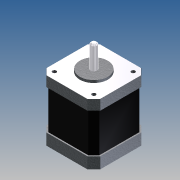
# Autodesk Inventor part: PM Wantai 811  Nema 17
Saved by Autodesk Inventor 2015 (Build 190159000, 159)
## iProperties
Created: 2013-09-15
Part Number: PM Wantai 811  Nema 17
Document SubType Name: Modeling
Designer: Phil
Density: 1 g/cm^3
Material: Generic
Appearance: Aluminum Cast
Author: Phil
Autodesk Inventor part; units mm, degrees
ref_plane "YZ Plane" through (0, 0, 0) normal (1, 0, 0) x (0, 1, 0)
ref_plane "XZ Plane" through (0, 0, 0) normal (0, 1, 0) x (-1, 0, 0)
sketch "Sketch1" plane through (0, 0, 0) normal (0, 0, 1) x (1, 0, 0)
  line L0 (-21.15, 21.15) -> (21.15, 21.15)
  line L1 (21.15, 21.15) -> (21.15, -21.15)
  line L2 (21.15, -21.15) -> (-21.15, -21.15)
  line L3 (-21.15, -21.15) -> (-21.15, 21.15)
  point P0 (0, 0)
  dimension "d0" = 42.3
  dimension "d1" = 42.3
  dimension "d2" = 21.15
  dimension "d3" = 21.15
  constraints: 8 end point, 2 parallel, 1 horizontal, 1 perpendicular
  measures "d0" distance between parallel lines of L2 L0
  measures "d1" distance of L1.end L2.end
  measures "d2" distance from line of L3 point (0, 0)
  measures "d3" distance from line of L2 point (0, 0)
extrude "Extrusion1" add sketch "Sketch1" along normal blind 48
sketch "Sketch2" plane through (0, 0, 48) normal (0, 0, 1) x (1, 0, 0)
  circle A0 centre (0, 0) radius 11
  dimension "d6" = 22
  constraints: 1 centre point, 1 coincident
  measures "d6" diameter of A0
extrude "Extrusion2" add sketch "Sketch2" along normal blind 2
sketch "Sketch3" plane through (0, 0, 50) normal (0, 0, 1) x (1, 0, 0)
  circle A0 centre (0, 0) radius 11 projected
  circle A1 centre (0, 0) radius 2.5
  dimension "d9" = 5
  constraints: 1 centre point, 1 coincident
  measures "d9" diameter of A1
extrude "Extrusion3" add sketch "Sketch3" along normal blind 18 contours A1
chamfer "Chamfer1" distance 5 angle 45 4 edges at (-21.15, 21.15, 24) (21.15, 21.15, 24) (-21.15, -21.15, 24) (21.15, -21.15, 24)
ref_plane "Work Plane1" through (0, 0, 40) normal (0, 0, 1) x (1, 0, 0)
sketch "Sketch4" plane through (0, 0, 40) normal (0, 0, 1) x (1, 0, 0)
  line L0 (21.15, -16.15) -> (16.15, -21.15) projected
  line L1 (21.15, 16.15) -> (21.15, -16.15) projected
  line L2 (16.15, 21.15) -> (21.15, 16.15) projected
  line L3 (-16.15, 21.15) -> (16.15, 21.15) projected
  line L4 (-21.15, 16.15) -> (-16.15, 21.15) projected
  line L5 (-21.15, -16.15) -> (-21.15, 16.15) projected
  line L6 (-16.15, -21.15) -> (-21.15, -16.15) projected
  line L7 (16.15, -21.15) -> (-16.15, -21.15) projected
  circle A0 centre (0, 0) radius 11 projected
  line L8 (15.7358, 20.15) -> (20.15, 15.7358)
  line L9 (20.15, 15.7358) -> (20.15, -15.7358)
  line L10 (20.15, -15.7358) -> (15.7358, -20.15)
  line L11 (15.7358, -20.15) -> (-15.7358, -20.15)
  line L12 (-15.7358, -20.15) -> (-20.15, -15.7358)
  line L13 (-20.15, -15.7358) -> (-20.15, 15.7358)
  line L14 (-20.15, 15.7358) -> (-15.7358, 20.15)
  line L15 (-15.7358, 20.15) -> (15.7358, 20.15)
  dimension "d16" = 1
  constraints: 16 end point, 7 other
  measures "d16" distance between parallel lines of L15 L3
extrude "Extrusion4" cut sketch "Sketch4" against normal blind 31 contours L0 L7 L6 L5 L4 L3 L2 L1
sketch "Sketch5" plane through (0, 0, 48) normal (0, 0, 1) x (1, 0, 0)
  line L0 (16.15, -21.15) -> (-16.15, -21.15) projected
  circle A0 centre (0, 0) radius 11 projected
  line L1 (0, 0) -> (0, 35.0575) construction
  line L2 (0, 0) -> (-35.907, 0) construction
  circle A1 centre (-15.5, 15.5) radius 1.5
  circle A2 centre (15.5, 15.5) radius 1.5
  circle A3 centre (-15.5, -15.5) radius 1.5
  circle A4 centre (15.5, -15.5) radius 1.5
  dimension "d19" = 3
  dimension "d20" = 15.5
  dimension "d21" = 15.5
  constraints: 4 centre point, 4 end point, 3 symmetric about line, 2 perpendicular, 3 other
  measures "d19" diameter of A1
  measures "d20" distance from line of L1 A1.centre
  measures "d21" distance from line of L2 A1.centre
extrude "Extrusion5" cut sketch "Sketch5" against normal blind 4 contours A1 | A2 | A3 | A4
fillet "Fillet1" radius 0.1 16 edges at (18.65, -18.65, 48) (21.15, 0, 48) (18.65, 18.65, 48) (0, 21.15, 48) (-18.65, 18.65, 48) (-21.15, 0, 48) (-18.65, -18.65, 48) (0, -21.15, 48) (18.65, -18.65, 0) (0, -21.15, 0) (-18.65, -18.65, 0) (-21.15, 0, 0) (-18.65, 18.65, 0) (0, 21.15, 0) (18.65, 18.65, 0) (21.15, 0, 0)
chamfer "Chamfer2" distance 1 angle 45 1 edges at (-2.5, 0, 68)
thread "Thread1" size "M3x0.5" class "6H" standard "ANSI Metric M Profile" full length
thread "Thread2" size "M3x0.5" class "6H" standard "ANSI Metric M Profile" full length
thread "Thread3" size "M3x0.5" class "6H" standard "ANSI Metric M Profile" full length
thread "Thread4" size "M3x0.5" class "6H" standard "ANSI Metric M Profile" full length
sketch "Sketch7" plane through (0, 0, 0) normal (0, 0, -1) x (-1, 0, 0)
  line L0 (0, 0) -> (30.0601, 0) construction
  line L1 (21.05, 16.1086) -> (21.05, -16.1086) projected
  line L2 (21.15, -16.15) -> (21.15, 16.15) projected
  line L3 (25.65, 8.15) -> (21.05, 8.15)
  line L4 (21.05, 8.15) -> (21.05, -8.15)
  line L5 (21.05, -8.15) -> (25.65, -8.15)
  line L6 (25.65, -8.15) -> (25.65, 8.15)
  dimension "d38" = 16.3
  dimension "d39" = 8.15
  dimension "d40" = 4.5
  constraints: 10 end point, 2 horizontal, 2 parallel, 1 perpendicular, 1 point on line
  measures "d38" distance between parallel lines of L5 L3
  measures "d39" distance between parallel lines of L0 L3
  measures "d40" distance between parallel lines of L2 L6
extrude "Extrusion7" add sketch "Sketch7" against normal blind 3
sketch "Sketch8" plane through (-21.15, -16.15, 9) normal (-1, 0, 0) x (0, 0, 1)
  line L0 (-6, 24.3) -> (-6, 8) projected
  line L1 (0, 0) -> (0, 32.3) projected
  line L2 (-6, 8) -> (0, 8)
  line L3 (0, 8) -> (0, 24.3)
  line L4 (0, 24.3) -> (-6, 24.3)
  line L5 (-6, 24.3) -> (-6, 8)
  line L6 (-8.9, 24.3) -> (-6, 24.3) projected
  point P0 (-9, 16.15)
  constraints: 8 end point, 2 collinear, 2 parallel, 1 horizontal, 1 perpendicular
extrude "Extrusion8" cut sketch "Sketch8" against normal blind 1
sketch "Sketch9" plane through (-20.15, -15.7358, 40) normal (-1, 0, 0) x (0, 0, 1)
  line L0 (-37, 7.5858) -> (-31, 7.5858)
  line L1 (-31, 7.5858) -> (-31, 23.8858)
  line L2 (-31, 23.8858) -> (-37, 23.8858)
  line L3 (-37, 23.8858) -> (-37, 7.5858)
  point P0 (-40, 15.7358)
  constraints: 8 end point, 2 parallel, 1 horizontal, 1 perpendicular
extrude "Extrusion9" add sketch "Sketch9" along normal blind 7
sketch "Sketch10" plane through (-27.15, -15.7358, 40) normal (-1, 0, 0) x (0, 0, 1)
  line L0 (-37, 7.5858) -> (-31, 7.5858) projected
  line L1 (-31, 7.5858) -> (-31, 23.8858) projected
  line L2 (-31, 23.8858) -> (-37, 23.8858) projected
  line L3 (-37, 23.8858) -> (-37, 7.5858) projected
  line L4 (-36.4, 8.1858) -> (-31.6, 8.1858)
  line L5 (-31.6, 8.1858) -> (-31.6, 23.2858)
  line L6 (-31.6, 23.2858) -> (-36.4, 23.2858)
  line L7 (-36.4, 23.2858) -> (-36.4, 8.1858)
  point P0 (-40, 15.7358)
  dimension "d47" = 0.6
  constraints: 8 end point, 3 other
  measures "d47" distance between parallel lines of L3 L7
extrude "Extrusion10" cut sketch "Sketch10" against normal blind 4.75 contours L7 L6 L5 L4
sketch "Sketch11" plane through (0, 0, 9) normal (0, 0, 1) x (1, 0, 0)
  line L0 (-20.15, 15.7358) -> (-20.15, -15.7358) projected
  line L1 (-15.7358, 20.15) -> (-20.15, 15.7358) projected
  line L2 (15.7358, 20.15) -> (-15.7358, 20.15) projected
  line L3 (20.15, 15.7358) -> (15.7358, 20.15) projected
  line L4 (20.15, -15.7358) -> (20.15, 15.7358) projected
  line L5 (15.7358, -20.15) -> (20.15, -15.7358) projected
  line L6 (-15.7358, -20.15) -> (15.7358, -20.15) projected
  line L7 (-20.15, -15.7358) -> (-15.7358, -20.15) projected
  line L8 (-21.15, 8.15) -> (-27.15, 8.15) projected
  line L9 (-27.15, -8.15) -> (-27.15, 8.15) projected
  line L10 (-21.15, -8.15) -> (-27.15, -8.15) projected
  line L11 (-21.15, -16.15) -> (-21.15, -8.15) projected
  line L12 (-16.15, -21.15) -> (-21.15, -16.15) projected
  line L13 (16.15, -21.15) -> (-16.15, -21.15) projected
  line L14 (21.15, -16.15) -> (16.15, -21.15) projected
  line L15 (21.15, 16.15) -> (21.15, -16.15) projected
  line L16 (16.15, 21.15) -> (21.15, 16.15) projected
  line L17 (-16.15, 21.15) -> (16.15, 21.15) projected
  line L18 (-21.15, 16.15) -> (-16.15, 21.15) projected
  line L19 (-21.15, 8.15) -> (-21.15, 16.15) projected
  line L20 (-27.15, -8.15) -> (-27.15, 8.15) projected
  line L21 (-27.15, 0) -> (-20.15, 0) construction
  line L22 (-20.15, 15.7358) -> (-20.15, -15.7358) projected
  line L23 (-27.15, -4) -> (-22.87, -4)
  line L24 (-22.87, -4) -> (-22.87, 4)
  line L25 (-22.87, 4) -> (-27.15, 4)
  line L26 (-27.15, 4) -> (-27.15, -4)
  point P0 (0, 0)
  dimension "d50" = 8
  dimension "d51" = 4
  dimension "d52" = 4.28
  constraints: 10 end point, 2 midpoint, 2 parallel, 1 horizontal, 1 perpendicular, 1 point on line
  measures "d50" distance between parallel lines of L25 L23
  measures "d51" distance between parallel lines of L21 L23
  measures "d52" distance between parallel lines of L24 L9
extrude "Extrusion11" cut sketch "Sketch11" against normal blind 1 contours L25 L24 L23 L9
sketch "Sketch12" plane through (-25.65, 8.15, 0) normal (0, 1, 0) x (1, 0, 0)
  line L0 (4.5, -0.1) -> (4.5, -9) projected
  line L1 (0, -3) -> (4.5, -3)
  line L2 (4.5, -3) -> (4.5, -3.1)
  line L3 (4.5, -3.1) -> (0, -3.1)
  line L4 (0, -3.1) -> (0, -3)
  point P0 (25.65, 0)
  dimension "d55" = 0.1
  constraints: 8 end point, 2 parallel, 1 horizontal, 1 perpendicular, 1 point on line
  measures "d55" distance between parallel lines of L1 L3
extrude "Extrusion12" cut sketch "Sketch12" against normal blind 0.1
mirror "Mirror1" about plane through (0, 0, 0) normal (0, 1, 0) of "Extrusion12"
sketch "Sketch13" plane through (0, 0, 9) normal (0, 0, 1) x (1, 0, 0)
  line L0 (-20.15, 15.7358) -> (-20.15, -15.7358) projected
  line L1 (-20.15, 8.15) -> (-20.15, 8.05)
  line L2 (-21.15, 8.15) -> (-21.15, 16.15) projected
  line L3 (-21.15, 8.2) -> (-20.15, 8.2)
  line L4 (-20.15, 8.2) -> (-20.15, 8.1)
  line L5 (-20.15, 8.1) -> (-21.15, 8.1)
  line L6 (-21.15, 8.1) -> (-21.15, 8.2)
  point P0 (0, 0)
  dimension "d61" = 0.1
  dimension "d62" = 0.05
  constraints: 10 end point, 3 point on line, 2 parallel, 1 horizontal, 1 perpendicular
  measures "d61" distance between parallel lines of L3 L5
  measures "d62" distance from line of L5 L2.start
extrude "Extrusion13" cut sketch "Sketch13" against normal blind 0.1
mirror "Mirror2" about plane through (0, 0, 0) normal (0, 1, 0) of "Extrusion13"
sketch "Sketch14" plane through (-22.4, -15.7358, 40) normal (-1, 0, 0) x (0, 0, 1)
  line L0 (-31.6, 8.1858) -> (-36.4, 8.1858) projected
  line L1 (-31.6, 23.2858) -> (-31.6, 8.1858) projected
  line L2 (-36.4, 23.2858) -> (-31.6, 23.2858) projected
  line L3 (-36.4, 8.1858) -> (-36.4, 23.2858) projected
  line L4 (-36.4, 8.1858) -> (-36.4, 23.2858) projected
  line L5 (-36.4, 15.7358) -> (-31.6, 15.7358) construction
  line L6 (-34.25, 14.4858) -> (-33.75, 14.4858)
  line L7 (-33.75, 14.4858) -> (-33.75, 14.9858)
  line L8 (-33.75, 14.9858) -> (-34.25, 14.9858)
  line L9 (-34.25, 14.9858) -> (-34.25, 14.4858)
  line L10 (-34, 15.7358) -> (-34, 8.6812) construction
  point P0 (-40, 15.7358)
  dimension "d63" = 0.75
  dimension "d64" = 0.5
  dimension "d65" = 0.25
  dimension "d66" = 0.5
  constraints: 12 end point, 3 midpoint, 2 horizontal, 2 parallel, 1 perpendicular, 1 vertical
  measures "d63" distance between parallel lines of L5 L8
  measures "d64" distance between parallel lines of L7 L9
  measures "d65" distance between parallel lines of L10 L9
  measures "d66" distance between parallel lines of L8 L6
extrude "Extrusion14" add sketch "Sketch14" along normal blind 4.6 contours L9 L8 L7 L6
chamfer "Chamfer3" distance 0.08 angle 70 4 edges at (-27, -1, 6.25) (-27, -0.75, 6) (-27, -1, 5.75) (-27, -1.25, 6) measured on face at (-27, -0.9167, 5.9167)
pattern_linear "Rectangular Pattern1" count 3 spacing 2.5 along (0, -1, 0) of "Extrusion14", "Chamfer3"
mirror "Mirror3" about plane through (0, 0, 0) normal (0, 1, 0) of "Extrusion14", "Chamfer3", "Rectangular Pattern1"
sketch "Sketch15" plane through (0, 0, 0) normal (0, 0, -1) x (-1, 0, 0)
  circle A0 centre (0, 0) radius 4.595
  dimension "d75" = 9.19
  constraints: 1 centre point, 1 coincident
  measures "d75" diameter of A0
extrude "Extrusion15" cut sketch "Sketch15" against normal blind 3.55
sketch "Sketch16" plane through (0, 0, 0) normal (0, 0, -1) x (-1, 0, 0)
  circle A0 centre (0, 0) radius 4.595 projected
  line L0 (21.05, 16.1086) -> (21.05, 8.15) projected
  line L1 (16.1086, 21.05) -> (21.05, 16.1086) projected
  line L2 (-16.1086, 21.05) -> (16.1086, 21.05) projected
  line L3 (-21.05, 16.1086) -> (-16.1086, 21.05) projected
  line L4 (-21.05, -16.1086) -> (-21.05, 16.1086) projected
  line L5 (-16.1086, -21.05) -> (-21.05, -16.1086) projected
  line L6 (16.1086, -21.05) -> (-16.1086, -21.05) projected
  line L7 (21.05, -16.1086) -> (16.1086, -21.05) projected
  line L8 (21.05, -8.15) -> (21.05, -16.1086) projected
  line L9 (21.05, -8.15) -> (25.65, -8.15) projected
  line L10 (25.65, -8.15) -> (25.65, 8.15) projected
  line L11 (25.65, 8.15) -> (21.05, 8.15) projected
  circle A1 centre (15, 15) radius 3
  dimension "d78" = 15
  dimension "d79" = 15
  dimension "d80" = 6
  constraints: 1 centre point
  measures "d78" horizontal distance of point (0, 0) A1.centre
  measures "d79" horizontal distance of point (0, 0) A1.centre
  measures "d80" diameter of A1
extrude "Extrusion16" cut sketch "Sketch16" against normal blind 2 contours A1
mirror "Mirror4" about plane through (0, 0, 0) normal (1, 0, 0) of "Extrusion16"
mirror "Mirror5" about plane through (0, 0, 0) normal (0, 1, 0) of "Extrusion16", "Mirror4"
sketch "Sketch17" plane through (-15, 15, 2) normal (0, 0, -1) x (-1, 0, 0)
  circle A0 centre (0, 0) radius 3 projected
  circle A1 centre (0, 0) radius 2.45
  point P0 (-15, -15)
  constraints: 1 centre point, 1 coincident
extrude "Extrusion17" add sketch "Sketch17" along normal blind 1.7 contours A1
sketch "Sketch18" plane through (-15, 15, 0.3) normal (0, 0, -1) x (-1, 0, 0)
  circle A0 centre (0, 0) radius 2.45 projected
  line L0 (1.5, 0.5) -> (-1.5, 0.5)
  line L1 (-1.5, 0.5) -> (-1.5, -0.5)
  line L2 (-1.5, -0.5) -> (1.5, -0.5)
  line L3 (1.5, -0.5) -> (1.5, 0.5)
  line L4 (0.5, 1.5) -> (-0.5, 1.5)
  line L5 (-0.5, 1.5) -> (-0.5, -1.5)
  line L6 (-0.5, -1.5) -> (0.5, -1.5)
  line L7 (0.5, -1.5) -> (0.5, 1.5)
  point P0 (-15, -15)
  dimension "d85" = 1
  dimension "d86" = 1
  dimension "d87" = 1.5
  dimension "d88" = 1.5
  dimension "d89" = 1.5
  dimension "d90" = 1.5
  dimension "d91" = 0.5
  dimension "d92" = 0.5
  constraints: 16 end point, 4 parallel, 2 horizontal, 2 perpendicular
  measures "d85" distance between parallel lines of L2 L0
  measures "d86" distance between parallel lines of L5 L7
  measures "d87" distance from line of A0.centre L4
  measures "d88" distance from line of A0.centre L6
  measures "d89" distance from line of A0.centre L3
  measures "d90" distance from line of L1 A0.centre
  measures "d91" distance from line of A0.centre L7
  measures "d92" distance from line of A0.centre L0
extrude "Extrusion18" cut sketch "Sketch18" against normal blind 0.6 contours L3 L2 L7 L0 | L7 L2 L5 L0 | L0 L5 L4 L7 | L5 L2 L1 L0 | L7 L6 L5 L2
fillet "Fillet2" radius 0.5 1 edges at (-12.55, 15, 0.3)
mirror "Mirror6" about plane through (0, 0, 0) normal (1, 0, 0) of "Extrusion17", "Extrusion18", "Fillet2"
mirror "Mirror7" about plane through (0, 0, 0) normal (0, 1, 0) of "Extrusion17", "Extrusion18", "Fillet2", "Mirror6"
sketch "Sketch19" plane through (0, 0, 3.55) normal (0, 0, -1) x (-1, 0, 0)
  circle A0 centre (0, 0) radius 2.5
  circle A1 centre (0, 0) radius 4.595 projected
  circle A2 centre (0, 0) radius 0.2846
  dimension "d96" = 5
  constraints: 2 centre point, 2 coincident
  measures "d96" diameter of A0
extrude "Extrusion19" add sketch "Sketch19" along normal blind 0.6 contours A0
chamfer "Chamfer4" distance 0.2 angle 45 1 edges at (2.5, 0, 2.95)
sketch "Sketch20" plane through (0, 0, 68) normal (0, 0, 1) x (1, 0, 0)
  circle A0 centre (0, 0) radius 2.5 projected
  line L0 (-7.2134, -5.8829) -> (-2, -5.8829)
  line L1 (-2, -5.8829) -> (-2, 8.324)
  line L2 (-2, 8.324) -> (-7.2134, 8.324)
  line L3 (-7.2134, 8.324) -> (-7.2134, -5.8829)
  dimension "d102" = 2
  constraints: 8 end point, 2 parallel, 1 horizontal, 1 perpendicular
  measures "d102" distance from line of L1 point (0, 0)
extrude "Extrusion20" cut sketch "Sketch20" against normal blind 17 contours L1 A0 | A0 L1 L0 L3 L2 picked at (-2.1667, 0)
equation "\"d1\" = d0"
equation "\"d2\" = 0.5 * d1"
equation "\"d3\" = 0.5 * d0"
equation "\"d20\" = d21"
equation "\"d39\" = 0.5 * d38"
equation "\"d51\" = 0.5 * d50"
equation "\"d65\" = 0.5 * d64"
equation "\"d66\" = d64"
equation "\"d79\" = d78"
equation "\"d86\" = d85"
equation "\"d88\" = d87"
equation "\"d89\" = d88"
equation "\"d90\" = d88"
equation "\"d91\" = 0.5 * d86"
equation "\"d92\" = 0.5 * d85"
body "Solid1"
